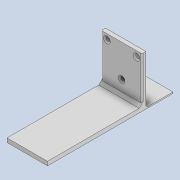
# Autodesk Inventor part: camera
Saved by Autodesk Inventor 2020 (Build 240168000, 168)
## iProperties
Created: 2022-02-18
Part Number: camera
Material: Типовые
Document SubType Name: Modeling
Designer: korra
Density: 1 g/cm^3
Appearance: По умолчанию
Author: korra
Autodesk Inventor part; units mm, degrees
ref_plane "YZ Plane" through (0, 0, 0) normal (1, 0, 0) x (0, 1, 0)
ref_plane "XZ Plane" through (0, 0, 0) normal (0, 1, 0) x (-1, 0, 0)
ref_plane "XY Plane" through (0, 0, 0) normal (0, 0, 1) x (1, 0, 0)
sketch "Эскиз1" plane through (0, 0, 0) normal (0, 0, 1) x (1, 0, 0)
  line L0 (0, 0) -> (-30, 0)
  line L1 (-30, 0) -> (-30, 38)
  line L2 (-30, 38) -> (0, 38)
  line L3 (0, 38) -> (0, 0)
  dimension "d0" = 30
  dimension "d1" = 38
  constraints: 8 end point, 2 parallel, 1 horizontal, 1 perpendicular
  measures "d0" distance of L1.end L2.end
  measures "d1" distance of L0.end L1.end
extrude "Выдавливание1" add sketch "Эскиз1" along normal blind 3
sketch "Эскиз2" plane through (0, 0, 0) normal (0, 0, -1) x (-1, 0, 0)
  line L0 (0, 0) -> (0, 38) projected
  line L1 (30, 38) -> (30, 0) projected
  line L2 (0, 0) -> (30, 0)
  line L3 (30, 0) -> (30, 2)
  line L4 (30, 2) -> (0, 2)
  line L5 (0, 2) -> (0, 0)
  point P0 (0, 2)
  dimension "d4" = 2
  constraints: 8 end point, 2 parallel, 1 horizontal, 1 perpendicular, 1 point on line
  measures "d4" distance between parallel lines of L2 L4
extrude "Выдавливание2" add sketch "Эскиз2" along normal blind 20
chamfer "Фаска1" distance 1 angle 45 1 edges at (-15, 2, 0)
sketch "Эскиз3" plane through (0, 0, 3) normal (0, 0, 1) x (1, 0, 0)
  circle A0 centre (-26, 34) radius 1.5
  circle A1 centre (-4, 34) radius 1.5
  circle A2 centre (-15, 14) radius 1.5
  line L0 (0, 38) -> (-30, 38) projected
  line L1 (-30, 38) -> (-30, 0) projected
  line L2 (0, 0) -> (0, 38) projected
  line L3 (-30, 0) -> (0, 0) projected
  dimension "d10" = 3
  dimension "d11" = 3
  dimension "d12" = 3
  dimension "d13" = 4
  dimension "d14" = 4
  dimension "d15" = 4
  dimension "d16" = 4
  dimension "d17" = 14
  dimension "d18" = 15
  constraints: 3 centre point
  measures "d10" diameter of A0
  measures "d11" diameter of A1
  measures "d12" diameter of A2
  measures "d13" distance from line of L0 A0.centre
  measures "d14" distance from line of L1 A0.centre
  measures "d15" distance from line of L0 A1.centre
  measures "d16" distance from line of L2 A1.centre
  measures "d17" distance from line of L3 A2.centre
  measures "d18" distance from line of L1 A2.centre
extrude "Выдавливание3" cut sketch "Эскиз3" against normal blind 20 contours A0 | A1 | A2
chamfer "Фаска2" distance 1 angle 45 3 edges at (-27.5, 34, 3) (-5.5, 34, 3) (-16.5, 14, 3)
sketch "Эскиз4" plane through (0, 0, 3) normal (0, 0, 1) x (1, 0, 0)
  line L0 (-30, 0) -> (-30, 2) projected
  line L1 (0, 0) -> (0, 38) projected
  line L2 (-30, 0) -> (0, 0)
  line L3 (0, 0) -> (0, 4)
  line L4 (0, 4) -> (-30, 4)
  line L5 (-30, 4) -> (-30, 0)
  dimension "d24" = 4
  constraints: 8 end point, 2 parallel, 1 horizontal, 1 perpendicular, 1 point on line
  measures "d24" distance between parallel lines of L2 L4
extrude "Выдавливание4" add sketch "Эскиз4" along normal blind 70
chamfer "Фаска3" distance 2 angle 45 1 edges at (-15, 4, 3)
chamfer "Фаска4" distance 1 angle 45 6 edges at (-30, 22, 3) (0, 22, 3) (-30, 0, 26.5) (-15, 0, 73) (0, 0, 26.5) (-15, 0, -20)
